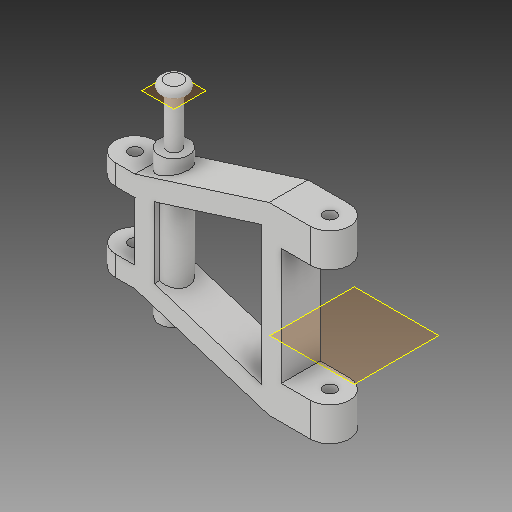
# Autodesk Inventor part: A_Arm
Saved by Autodesk Inventor 2019 (Build 230136000, 136)
## iProperties
Created: 2019-03-03
Part Number: A_Arm
Material: Generic
Document SubType Name: Modeling
Designer: alarr
Density: 1 g/cm^3
Appearance: Default
Author: alarr
Autodesk Inventor part; units mm, degrees
ref_plane "YZ Plane" through (0, 0, 0) normal (1, 0, 0) x (0, 1, 0)
ref_plane "XZ Plane" through (0, 0, 0) normal (0, 1, 0) x (-1, 0, 0)
ref_plane "XY Plane" through (0, 0, 0) normal (0, 0, 1) x (1, 0, 0)
ref_plane "Work Plane1" through (0, -15.24, 5.08) normal (0, 1, 0) x (-1, 0, 0)
sketch "Sketch2" plane through (0, -15.24, 0) normal (0, 1, 0) x (-1, 0, 0)
  arc A0 (6.35, -5.08) -> (6.35, 5.08) centre (6.35, 0) ccw construction
  line L0 (6.35, 5.08) -> (0, 5.08) projected
  line L1 (0, -5.08) -> (6.35, -5.08) projected
  circle A1 centre (6.35, 0) radius 1.5875 projected
  arc A2 (6.35, 5.08) -> (6.35, -5.08) centre (6.35, 0) ccw
  line L2 (6.35, 5.08) -> (57.15, 5.08)
  line L3 (6.35, -5.08) -> (57.15, -5.08)
  arc A3 (57.15, -5.08) -> (57.15, 5.08) centre (57.15, 0) ccw
  arc A4 (6.35, -5.08) -> (6.35, 5.08) centre (6.35, 0) ccw construction
  arc A5 (57.15, 5.08) -> (57.15, -5.08) centre (57.15, 0) ccw construction
  point P0 (0, 0)
  dimension "d0" = 50.8
  constraints: 8 point on circle, 6 tangent, 4 centre point, 4 end point, 2 horizontal, 1 coincident, 1 concentric
  measures "d0" distance of L0.start L2.end
extrude "Extrusion1" add sketch "Sketch2" along normal mid plane 48.006
sketch "Sketch3" plane through (-57.15, 8.763, 5.08) normal (0, 0, 1) x (1, 0, 0)
  line L0 (57.15, -8.763) -> (57.15, -39.243) projected
  line L1 (50.8, -8.763) -> (57.15, -8.763) projected
  line L2 (50.8, -8.763) -> (50.8, -39.243) projected
  line L3 (57.15, -39.243) -> (50.8, -39.243) projected
  line L4 (55.88, -48.006) -> (55.88, 0) projected
  line L5 (55.88, -39.243) -> (55.88, -8.763)
  line L6 (55.88, -8.763) -> (43.18, -8.763)
  line L7 (43.18, -8.763) -> (43.18, -39.243)
  line L8 (5.08, -11.049) -> (40.005, 0)
  line L9 (50.8, 0) -> (0, 0) projected
  line L10 (0, -48.006) -> (0, 0) construction
  line L11 (0, 0) -> (0, 0) projected
  line L12 (0, -48.006) -> (0, 0) construction
  line L13 (0, -48.006) -> (0, -48.006) projected
  line L14 (40.005, 0) -> (55.88, 0) construction
  line L15 (55.88, -24.003) -> (-5.08, -24.003) construction
  line L16 (40.005, 0) -> (-5.08, 0)
  line L17 (-5.08, -11.049) -> (-5.08, 0)
  line L18 (5.08, -36.957) -> (40.005, -48.006)
  line L19 (5.08, -36.957) -> (-5.08, -36.957)
  line L20 (40.005, -48.006) -> (55.88, -48.006) construction
  line L21 (50.8, -48.006) -> (0, -48.006) projected
  line L22 (-5.08, -48.006) -> (0, -48.006) projected
  line L23 (-5.08, -48.006) -> (-5.08, 0) construction
  line L24 (40.005, -48.006) -> (-5.08, -48.006)
  line L25 (-5.08, -36.957) -> (-5.08, -48.006)
  line L26 (0, -48.006) -> (0, 0) construction
  line L27 (5.08, -11.049) -> (-5.08, -11.049)
  line L28 (5.08, -36.957) -> (5.08, -11.049) construction
  line L29 (55.88, -39.243) -> (43.18, -39.243)
  dimension "d3" = 15.875
  dimension "d5" = 25.908
  dimension "d10" = 10.16
  dimension "d17" = 12.7
  constraints: 32 end point, 4 horizontal, 4 point on line, 3 perpendicular, 2 midpoint, 2 symmetric about line, 1 collinear, 1 parallel
  measures "d3" distance from line of L8.end L4
  measures "d5" distance between parallel lines of L19 L27
  measures "d10" distance between parallel lines of L23 L28
  measures "d17" distance between parallel lines of L7 L4
extrude "Extrusion2" cut sketch "Sketch3" against normal through all
sketch "Sketch4" plane through (-57.15, -2.286, 0) normal (0, 1, 0) x (1, 0, 0)
  arc A0 (0, 5.08) -> (0, -5.08) centre (0, 0) ccw projected
  circle A1 centre (0, 0) radius 1.5875
  circle A2 centre (50.8, 0) radius 1.5875 projected
  point P0 (57.15, 0)
  constraints: 1 centre point, 1 coincident, 1 equal radius
extrude "Extrusion3" cut sketch "Sketch4" against normal through all contours A1
sketch "Sketch6" plane through (-17.145, -39.243, 5.08) normal (0, 0, 1) x (1, 0, 0)
  line L0 (-45.085, 11.049) -> (-45.085, 36.957) projected
  line L1 (-40.005, 11.049) -> (-45.085, 11.049) projected
  line L2 (-40.005, 11.049) -> (-34.925, 11.049) projected
  line L3 (-45.085, 36.957) -> (-40.005, 36.957) projected
  line L4 (-34.925, 36.957) -> (-40.005, 36.957) projected
  line L5 (-45.085, 31.623) -> (-34.925, 31.623)
  line L6 (-34.925, 31.623) -> (-34.925, 16.383)
  line L7 (-34.925, 16.383) -> (-45.085, 16.383)
  line L8 (-45.085, 16.383) -> (-45.085, 31.623)
  line L9 (-45.085, 31.623) -> (-34.925, 16.383) construction
  line L10 (-34.925, 31.623) -> (-45.085, 16.383) construction
  line L11 (-40.005, 24.003) -> (-45.085, 24.003) construction
  point P0 (17.145, 39.243)
  dimension "d19" = 10.16
  dimension "d20" = 15.24
  constraints: 14 end point, 4 midpoint, 2 parallel, 1 horizontal, 1 perpendicular
  measures "d19" distance between parallel lines of L0 L6
  measures "d20" distance between parallel lines of L5 L7
extrude "Extrusion5" cut sketch "Sketch6" against normal through all
sketch "Sketch5" plane through (-17.145, -39.243, 5.08) normal (0, 0, 1) x (1, 0, 0)
  line L0 (-40.005, 11.049) -> (-34.925, 11.049) projected
  line L1 (-34.925, 11.049) -> (0, 0) projected
  line L2 (10.795, 0) -> (0, 0) projected
  line L3 (10.795, 0) -> (10.795, 8.763) projected
  line L4 (10.795, 39.243) -> (10.795, 48.006) projected
  line L5 (0, 48.006) -> (10.795, 48.006) projected
  line L6 (0, 48.006) -> (-34.925, 36.957) projected
  line L7 (-34.925, 36.957) -> (-40.005, 36.957) projected
  line L8 (-40.005, 11.049) -> (-40.005, 16.383) projected
  line L9 (10.795, 8.763) -> (3.175, 8.763) projected
  line L10 (3.175, 8.763) -> (3.175, 39.243) projected
  line L11 (3.175, 39.243) -> (10.795, 39.243) projected
  line L12 (-40.005, 31.623) -> (-34.925, 31.623) projected
  line L13 (-34.925, 31.623) -> (-34.925, 16.383) projected
  line L14 (-34.925, 16.383) -> (-40.005, 16.383) projected
  line L15 (-40.005, 31.623) -> (-40.005, 36.957) projected
  line L16 (-1.905, 5.9308) -> (-29.845, 14.77)
  line L17 (-29.845, 14.77) -> (-29.845, 33.236)
  line L18 (-29.845, 33.236) -> (-1.905, 42.0752)
  line L19 (-1.905, 42.0752) -> (-1.905, 5.9308)
  dimension "d23" = 5.08
  constraints: 8 end point, 3 other
  measures "d23" distance between parallel lines of L1 L16
extrude "Extrusion4" cut sketch "Sketch5" against normal through all contours L16 L17 L18 L19
sketch "Sketch8" plane through (0, -15.24, 5.08) normal (0, 1, 0) x (-1, 0, 0)
  circle A0 centre (46.99, -5.08) radius 3.81
  arc A1 (57.15, -10.16) -> (57.15, 0) centre (57.15, -5.08) ccw projected
  line L0 (62.23, -5.08) -> (46.99, -5.08) construction
  point P0 (0, -5.08)
  dimension "d24" = 7.62
  dimension "d25" = 15.24
  constraints: 2 end point, 1 centre point, 1 horizontal, 1 point on circle, 1 point on line
  measures "d24" diameter of A0
  measures "d25" distance of L0.start L0.end
extrude "Extrusion6" add sketch "Sketch8" along normal mid plane 38.1
sketch "Sketch9" plane through (-46.99, 3.81, 0) normal (0, 1, 0) x (1, 0, 0)
  circle A0 centre (0, 0) radius 1.8415
  circle A1 centre (0, 0) radius 3.81 projected
  point P0 (46.99, 0)
  dimension "d28" = 3.683
  constraints: 1 centre point, 1 coincident
  measures "d28" diameter of A0
extrude "Extrusion7" cut sketch "Sketch9" against normal through all contours A0
ref_plane "Work Plane2" through (-46.99, 16.51, 0) normal (0, 1, 0) x (1, 0, 0)
sketch "Sketch10" plane through (-46.99, 16.51, 0) normal (0, 1, 0) x (1, 0, 0)
  circle A0 centre (0, 0) radius 1.8415 projected
  circle A1 centre (0, 0) radius 1.8415
  point P0 (46.99, 0)
  constraints: 1 centre point, 1 coincident, 1 concentric
extrude "Extrusion8" add sketch "Sketch10" against normal up to surface (44.704 mm away)
sketch "Sketch11" plane through (-46.99, 16.51, 0) normal (0, 1, 0) x (1, 0, 0)
  circle A0 centre (0, 0) radius 3.81 projected
  circle A1 centre (0, 0) radius 3.4925
  point P0 (46.99, 0)
  dimension "d34" = 6.985
  constraints: 1 centre point, 1 coincident
  measures "d34" diameter of A1
extrude "Extrusion9" add sketch "Sketch11" along normal blind 2.54 contours A1
full round fillet "Fillet1" first side at (-44.0995, 16.51, 0.4255) centre faces at (-43.5088, 18.2033, 0.281) second side at (-46.6012, 19.05, -0.8909)
body "Solid1"
